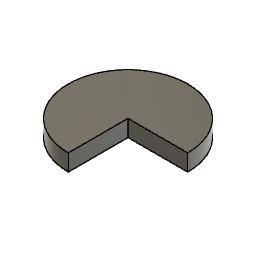
Corner Helper v1 (Autodesk Fusion 360 design; units mm, degrees)
Autodesk Fusion 360 part; units mm, degrees
sketch "Sketch1" plane through (0, 0, 0) normal (0, 1, 0) x (1, 0, 0)
  line L0 (0, 0) -> (9, 0)
  line L1 (0, -9) -> (0, 0)
  arc A0 (9, 0) -> (0, -9) centre (0, 0) ccw
  dimension "d1" = 18
  constraint coincident L0.start L1.end
  constraint horizontal L0
  constraint vertical L1
  measures "d1" diameter of A0
extrude "Extrude1" add sketch "Sketch1" along normal blind 2.5
